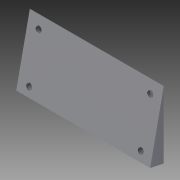
# Autodesk Inventor part: Third_Flame_Spacer
Saved by Autodesk Inventor 2013 (Build 170138000, 138)
## iProperties
Created: 2014-04-17
Part Number: Third_Flame_Spacer
Material: アセタール樹脂、白
Document SubType Name: Modeling
Designer: andou
Density: 1 g/cm^3
Author: andou
Autodesk Inventor part; units mm, degrees
ref_plane "YZ Plane" through (0, 0, 0) normal (1, 0, 0) x (0, 1, 0)
ref_plane "XZ Plane" through (0, 0, 0) normal (0, 1, 0) x (-1, 0, 0)
ref_plane "XY Plane" through (0, 0, 0) normal (0, 0, 1) x (1, 0, 0)
sketch "スケッチ1" plane through (0, 0, 0) normal (1, 0, 0) x (0, 1, 0)
  line L0 (2, 15) -> (2, -15)
  line L1 (2, -15) -> (-4.101, -13.7032)
  line L2 (-4.101, -13.7032) -> (2, 15)
  point P0 (0, 0)
  dimension "d0" = 12
  dimension "d1" = 30
  dimension "d4" = 2
  dimension "d5" = 15
  constraints: 6 end point, 1 perpendicular, 1 vertical
  measures "d0" angle of L0 L2
  measures "d1" distance of L0.start L0.end
  measures "d4" distance from line of L0 point (0, 0)
  measures "d5" vertical distance of L0.end point (0, 0)
extrude "押し出し1" add sketch "スケッチ1" along normal blind 60
sketch "スケッチ2" plane through (0, 2, 15) normal (0, 1, 0) x (1, 0, 0)
  line L0 (60, 30) -> (60, 0) projected
  line L1 (0, 30) -> (60, 30) projected
  circle A0 centre (5, 5) radius 1.3
  circle A1 centre (5, 25) radius 1.3
  circle A2 centre (55, 5) radius 1.3
  circle A3 centre (55, 25) radius 1.3
  point P0 (0, 15)
  dimension "d8" = 2.6
  dimension "d11" = 50
  dimension "d12" = 50
  dimension "d13" = 20
  dimension "d14" = 20
  dimension "d15" = 5
  dimension "d16" = 5
  dimension "d17" = 5
  dimension "d18" = 5
  constraints: 4 centre point, 3 equal radius
  measures "d8" diameter of A1
  measures "d11" distance of A3.centre A1.centre
  measures "d12" distance of A2.centre A0.centre
  measures "d13" distance of A3.centre A2.centre
  measures "d14" distance of A0.centre A1.centre
  measures "d15" distance from line of L1 A1.centre
  measures "d16" distance from line of L1 A3.centre
  measures "d17" distance from line of L0 A2.centre
  measures "d18" distance from line of L0 A3.centre
hole "穴1" at (5, 2, 10) at (55, 2, 10) at (55, 2, -10) at (5, 2, -10) direction (0, -1, 0) diameter 2.6 end through all
thread "ねじ1" size "M2.6x0.45" class "6H" standard "ANSI Metric M Profile" full length
thread "ねじ2" size "M2.6x0.45" class "6H" standard "ANSI Metric M Profile" full length
thread "ねじ3" size "M2.6x0.45" class "6H" standard "ANSI Metric M Profile" full length
thread "ねじ4" size "M2.6x0.45" class "6H" standard "ANSI Metric M Profile" full length
